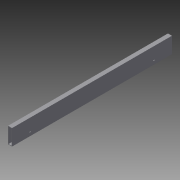
# Autodesk Inventor part: 4x1 boxbeam
Saved by Autodesk Inventor 2015 (Build 190159000, 159)
## iProperties
Created: 2015-01-11
Part Number: 4x1 boxbeam
Material: Generic
Document SubType Name: Modeling
Designer: chapale16
Density: 1 g/cm^3
Appearance: Default
Author: chapale16
Autodesk Inventor part; units mm, degrees
ref_plane "YZ Plane" through (0, 0, 0) normal (1, 0, 0) x (0, 1, 0)
ref_plane "XZ Plane" through (0, 0, 0) normal (0, 1, 0) x (-1, 0, 0)
ref_plane "XY Plane" through (0, 0, 0) normal (0, 0, 1) x (1, 0, 0)
sketch "Sketch1" plane through (0, 0, 0) normal (0, 0, 1) x (1, 0, 0)
  line L0 (0, 0) -> (25.4, 0)
  line L1 (25.4, 0) -> (25.4, -101.6)
  line L2 (25.4, -101.6) -> (0, -101.6)
  line L3 (0, -101.6) -> (0, 0)
  line L4 (22.225, -3.175) -> (3.175, -3.175)
  line L5 (3.175, -3.175) -> (3.175, -98.425)
  line L6 (3.175, -98.425) -> (22.225, -98.425)
  line L7 (22.225, -98.425) -> (22.225, -3.175)
  dimension "d0" = 25.4
  dimension "d1" = 101.6
  dimension "d2" = 3.175
  constraints: 16 end point, 4 parallel, 2 perpendicular, 1 horizontal, 3 other
  measures "d0" distance of L1.end L2.end
  measures "d1" distance of L0.end L1.end
  measures "d2" distance between parallel lines of L0 L4
extrude "Extrusion1" add sketch "Sketch1" along normal blind 1016
sketch "Sketch2" plane through (25.4, -101.6, 0) normal (1, 0, 0) x (0, 0, -1)
  point P0 (0, 101.6)
  point P1 (-114.3, 25.4)
sketch "Sketch3" plane through (25.4, -101.6, 0) normal (1, 0, 0) x (0, 0, -1)
  point P0 (0, 101.6)
  point P1 (-901.7, 25.4)
hole "Hole1" at (25.4, -76.2, 901.7) direction (-1, 0, 0) diameter 9.525 end through all
hole "Hole2" at (25.4, -76.2, 114.3) direction (-1, 0, 0) diameter 9.525 end through all
body "Solid1"
